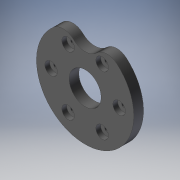
# Autodesk Inventor part: AA033
Saved by Autodesk Inventor 2017 SP1 (Build 210196100, 196)
## iProperties
Created: 2017-10-14
Part Number: AA033
Material: ABS Plastic
Document SubType Name: Modeling
Designer: Zach
Density: 1.06 g/cm^3
Appearance: CR White
Author: Zach
Autodesk Inventor part; units mm, degrees
ref_plane "YZ Plane" through (0, 0, 0) normal (1, 0, 0) x (0, 1, 0)
ref_plane "XZ Plane" through (0, 0, 0) normal (0, 1, 0) x (-1, 0, 0)
ref_plane "XY Plane" through (0, 0, 0) normal (0, 0, 1) x (1, 0, 0)
sketch "Sketch1" plane through (0, 0, 0) normal (0, 0, 1) x (1, 0, 0)
  circle A0 centre (0, 0) radius 50
  circle A1 centre (0, 0) radius 16.5
  circle A2 centre (35, 0) radius 2.5
  circle A3 centre (17.5, 30.3109) radius 2.5
  circle A4 centre (-17.5, 30.3109) radius 2.5
  circle A5 centre (-35, 0) radius 2.5
  circle A6 centre (-17.5, -30.3109) radius 2.5
  circle A7 centre (17.5, -30.3109) radius 2.5
  dimension "d0" = 100
  dimension "d1" = 33
  dimension "d2" = 5
  dimension "d3" = 35
  dimension "d6" = 360
  constraints: 8 centre point, 2 coincident, 1 horizontal alignment, 13 other
  measures "d0" diameter of A0
  measures "d1" diameter of A1
  measures "d2" diameter of A2
  measures "d3" distance of A2.centre point (0, 0)
extrude "Extrusion1" add sketch "Sketch1" along normal blind 10
sketch "Sketch2" plane through (0, 0, 10) normal (0, 0, 1) x (1, 0, 0)
  circle A0 centre (35, 0) radius 2.5 projected
  circle A1 centre (35, 0) radius 6.5
  circle A2 centre (17.5, 30.3109) radius 6.5
  circle A3 centre (-17.5, 30.3109) radius 6.5
  circle A4 centre (-35, 0) radius 6.5
  circle A5 centre (-17.5, -30.3109) radius 6.5
  circle A6 centre (17.5, -30.3109) radius 6.5
  point P0 (0, 0)
  dimension "d10" = 13
  dimension "d13" = 360
  constraints: 6 centre point, 6 coincident, 19 other
  measures "d10" diameter of A1
extrude "Extrusion2" cut sketch "Sketch2" against normal blind 5 contours A0 | A1 | A2 | A3 | A4 | A5 | A6
sketch "Sketch3" plane through (0, 0, 10) normal (0, 0, 1) x (1, 0, 0)
  circle A0 centre (0, 0) radius 50 construction
  circle A1 centre (0, 50) radius 17.5
  dimension "d17" = 35
  constraints: 2 vertical alignment, 1 centre point, 1 other
  measures "d17" diameter of A1
extrude "Extrusion3" cut sketch "Sketch3" against normal through all
fillet "Fillet1" radius 15 2 edges at (-17.2299, 46.9375, 5) (17.2299, 46.9375, 5)
body "Solid1"
